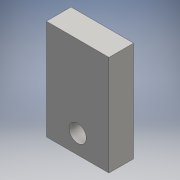
# Autodesk Inventor part: StupidPiece
Saved by Autodesk Inventor 2016 (Build 200138000, 138)
## iProperties
Created: 2017-03-11
Part Number: StupidPiece
Material: Generic
Document SubType Name: Modeling
Designer: Owner
Density: 1 g/cm^3
Appearance: Default
Author: Owner
Autodesk Inventor part; units mm, degrees
ref_plane "YZ Plane" through (0, 0, 0) normal (1, 0, 0) x (0, 1, 0)
ref_plane "XZ Plane" through (0, 0, 0) normal (0, 1, 0) x (-1, 0, 0)
ref_plane "XY Plane" through (0, 0, 0) normal (0, 0, 1) x (1, 0, 0)
sketch "Sketch1" plane through (0, 0, 0) normal (0, 1, 0) x (-1, 0, 0)
  line L0 (12.7, -214.55) -> (12.7, -224.71)
  line L1 (12.7, -224.71) -> (0, -224.71)
  line L2 (0, -224.71) -> (0, -214.55)
  line L3 (0, -214.55) -> (12.7, -214.55)
  line L4 (12.7, -214.55) -> (12.7, -224.71)
  circle A0 centre (6.35, -220.9) radius 1.75
  circle A1 centre (6.35, -220.9) radius 1.75
  point P0 (0, 0)
  constraints: 10 end point, 2 centre point, 2 parallel, 1 coincident, 1 horizontal, 1 perpendicular
extrude "Extrusion1" add sketch "Sketch1" along normal blind 5.0038
sketch "Sketch2" plane through (-12.7, 0, -214.55) normal (0, 0, 1) x (1, 0, 0)
  line L0 (12.7, 0) -> (0, 0) projected
  line L1 (12.7, 0) -> (12.7, 5.0038) projected
  line L2 (0, 5.0038) -> (12.7, 5.0038) projected
  line L3 (0, 0) -> (0, 5.0038) projected
extrude "Extrusion2" add sketch "Sketch2" along normal blind 10.16
body "Solid1"
